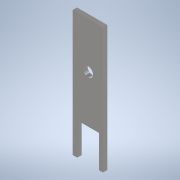
# Autodesk Inventor part: backWheelNoMotor brake mount
Saved by Autodesk Inventor 2022.2 (Build 262287010, 287A)
## iProperties
Created: 2022-04-04
Part Number: backWheelNoMotor brake mount
Material: Steel, Mild
Document SubType Name: Sheet Metal
Designer: foriw
Density: 7.85 g/cm^3
Sheet Metal Rule: Default_mm
Appearance: Semi-Polished
Author: foriw
Autodesk Inventor part; units mm, degrees
ref_plane "YZ Plane" through (0, 0, 0) normal (1, 0, 0) x (0, 1, 0)
ref_plane "XZ Plane" through (0, 0, 0) normal (0, 1, 0) x (-1, 0, 0)
ref_plane "XY Plane" through (0, 0, 0) normal (0, 0, 1) x (1, 0, 0)
sketch "Sketch1" plane through (0, 0, 0) normal (0, 0, 1) x (1, 0, 0)
  line L0 (0, 57.8309) -> (-14, 57.8309) projected
  line L1 (0, 0) -> (-14, 0)
  line L2 (-14, 0) -> (-14, 57.8309)
  line L3 (-14, 57.8309) -> (0, 57.8309)
  line L4 (0, 57.8309) -> (0, 0)
  line L5 (-14, 57.8309) -> (0, 57.8309)
  line L6 (0, 57.8309) -> (0, 77.8309)
  line L7 (0, 77.8309) -> (-14, 77.8309)
  line L8 (-14, 77.8309) -> (-14, 57.8309)
  line L9 (0, 0) -> (0, -4)
  line L10 (0, -4) -> (-14, -4)
  line L11 (-14, 0) -> (-14, -4)
  dimension "d0" = 20
  dimension "d7" = 4
  constraints: 22 end point, 4 parallel, 3 perpendicular, 2 horizontal, 2 vertical, 1 point on line
  measures "d0" distance of L6.end L5.end
  measures "d7" distance of L1.start L9.end
extrude "Extrusion1" add sketch "Sketch1" along normal blind 2 contours L4 L1 L2 L0
sketch "Sketch2" plane through (0, 0, 2) normal (0, 0, 1) x (1, 0, 0)
  circle A0 centre (-5.7096, 36.7123) radius 6.15 projected
  circle A1 centre (-5.7096, 36.7123) radius 2.15 projected
  circle A2 centre (-6.8781, 4.5836) radius 17.5 projected
  circle A3 centre (-6.8781, 4.5836) radius 5 projected
  circle A4 centre (-6.8781, 4.5836) radius 32.15
  circle A5 centre (-6.8781, 36.7336) radius 2.25
  line L0 (-6.8781, 4.5836) -> (-6.8781, 17.8952) construction
  line L1 (-6.8781, 36.7336) -> (-6.8781, 4.5836) construction
  line L2 (-11.8781, -0.9531) -> (-11.8781, 14.8638)
  line L3 (-11.8781, 14.8638) -> (-1.8781, 14.8638)
  line L4 (-1.8781, 14.8638) -> (-1.8781, -0.9531)
  line L5 (-1.8781, -0.9531) -> (-11.8781, -0.9531)
  arc A6 (-1.8781, 4.5836) -> (-11.8781, 4.5836) centre (-6.8781, 4.5836) ccw projected
  arc A7 (-1.8781, 4.5836) -> (-11.8781, 4.5836) centre (-6.8781, 4.5836) ccw projected
  point P0 (0, 0)
  point P1 (-1.8781, 4.5836)
  point P2 (-11.8781, 4.5836)
  dimension "d3" = 4.5
  dimension "d4" = 0
  constraints: 12 end point, 2 centre point, 2 point on circle, 2 tangent, 2 vertical, 1 coincident, 1 perpendicular
  measures "d3" diameter of A5
  measures "d4" distance between parallel lines of L1 L0
extrude "Extrusion2" cut sketch "Sketch2" against normal through all contours A5 A1 A4 | A4 A1 A5 | A4 A5 A1 | A1 A5 A4 | A3 | L4 L5 L2 A3 | A3 L2 L3 L4 picked at (-8.3259, 37.2162) picked at (-8.3126, 36.1952) picked at (-6.3657, 36.0685) picked at (-6.3452, 37.3793)
equation "\"BendRadius\" = Thickness"
equation "\"BendReliefWidth\" = Thickness"
equation "\"BendReliefDepth\" = 0.5 * Thickness"
equation "\"CornerReliefSize\" = 4 * Thickness"
equation "\"MinimumRemnant\" = 2 * Thickness"
equation "\"TransitionRadius\" = BendRadius"
equation "\"JacobiRadiusSize\" = BendRadius"
equation "\"GapSize\" = Thickness"
equation "\"Thickness\" = 2"
body "Solid1"
